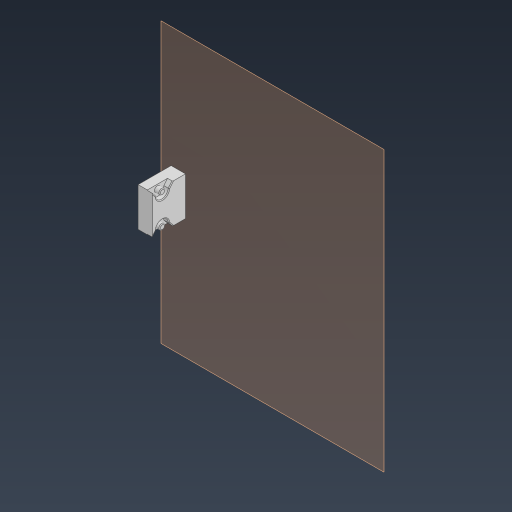
# Autodesk Inventor part: front-lunad-holder
Saved by Autodesk Inventor 2023 (Build 270158000, 158)
## iProperties
Created: 2025-04-06
Part Number: front-lunad-holder
Material: Generic
Document SubType Name: Modeling
Designer: szymo
Density: 1 g/cm^3
Appearance: Default
Author: szymo
Autodesk Inventor part; units mm, degrees
ref_plane "YZ Plane" through (0, 0, 0) normal (1, 0, 0) x (0, 1, 0)
ref_plane "XZ Plane" through (0, 0, 0) normal (0, 1, 0) x (-1, 0, 0)
ref_plane "XY Plane" through (0, 0, 0) normal (0, 0, 1) x (1, 0, 0)
ref_plane "Work Plane1" through (0, 0, 0) normal (0, 0, 1) x (1, 0, 0)
sketch "Sketch1" plane through (0, 0, 0) normal (0, 0, 1) x (1, 0, 0)
  line L0 (-33.9, 7.85) -> (-44.9, 7.85) projected
  line L1 (-35.9, 5.925) -> (-35.9, 7.85) projected
  line L2 (-35.9, 5.925) -> (-35.9, 3.675) projected
  line L3 (-35.9, -7.85) -> (-35.9, -5.925) projected
  line L4 (-35.9, -3.675) -> (-35.9, -5.925) projected
  line L5 (-44.9, -7.85) -> (-33.9, -7.85) projected
  line L6 (-33.9, 7.55) -> (-44.9, 7.55)
  line L7 (-44.9, -7.55) -> (-33.9, -7.55)
  line L8 (-39.5, 49.5) -> (-39.5, -49.5) projected
  line L9 (-39.5, 7.55) -> (-39.5, -7.55)
  line L10 (-33.9, 5.925) -> (-33.9, 3.675) projected
  line L11 (-33.9, 5.925) -> (-33.9, 7.85) projected
  line L12 (-35.9, 3.675) -> (-33.9, 3.675)
  line L13 (-33.9, -7.85) -> (-33.9, -5.925) projected
  line L14 (-33.9, -3.675) -> (-33.9, -5.925) projected
  line L15 (-35.9, -3.675) -> (-33.9, -3.675)
  line L16 (-33.9, 3.675) -> (-33.9, -3.675)
  line L17 (-35.9, -3.675) -> (-35.9, 3.675)
  point P0 (0, 0)
  dimension "d0" = 0.3
  dimension "d1" = 0.3
  constraints: 14 end point, 4 point on line, 3 parallel, 2 horizontal, 1 collinear
  measures "d0" distance between parallel lines of L0 L6
  measures "d1" distance between parallel lines of L5 L7
extrude "Extrusion1" add sketch "Sketch1" along normal up to surface (12.8653 mm away) contours L11 L10 L12 L2 L1 L6 | L1 L2 L17 L4 L3 L7 L8 L6 | L16 L15 L17 L12 | L14 L13 L7 L3 L4 L15
sketch "Sketch2" plane through (-33.9, -7.55, 0) normal (1, 0, 0) x (0, 0, -1)
  arc A0 (-6.75, 1.625) -> (-11.25, 1.625) centre (-9, 1.625) ccw projected
  line L0 (-12.8653, -0.3) -> (-11.25, 1.625) projected
  line L1 (-6.75, 1.625) -> (-5.1347, -0.3) projected
  line L2 (-5.1347, 15.4) -> (-6.75, 13.475) projected
  arc A1 (-11.25, 13.475) -> (-6.75, 13.475) centre (-9, 13.475) ccw projected
  line L3 (-11.25, 13.475) -> (-12.8653, 15.4) projected
  line L4 (-12.8653, 15.1) -> (-12.8653, 0) projected
  line L5 (0, 0) -> (-12.8653, 0) projected
  line L6 (0, 0) -> (0, 15.1) projected
  line L7 (0, 15.1) -> (-12.8653, 15.1) projected
  line L8 (-13.0951, -0.1072) -> (-11.5475, 1.7371)
  arc A2 (-6.4525, 1.7371) -> (-11.5475, 1.7371) centre (-9, 1.625) ccw
  line L9 (-6.4525, 1.7371) -> (-4.9049, -0.1072)
  line L10 (-4.9049, 15.2072) -> (-6.4525, 13.3629)
  arc A3 (-11.5475, 13.3629) -> (-6.4525, 13.3629) centre (-9, 13.475) ccw
  line L11 (-11.5475, 13.3629) -> (-13.0951, 15.2072)
  circle A4 centre (-9, 1.625) radius 1.1 projected
  circle A5 centre (-9, 13.475) radius 1.1 projected
  circle A6 centre (-9, 1.625) radius 1
  circle A7 centre (-9, 13.475) radius 1
  point P0 (0, 7.55)
  point P1 (-12.8653, 14.9333)
  point P2 (-4.9948, 15.1)
  point P3 (-4.9948, 0)
  point P4 (-12.8653, 0.1667)
  dimension "d4" = 0.3
  dimension "d5" = 0.3
  dimension "d6" = 0.1
  dimension "d7" = 0.1
  constraints: 8 end point, 4 centre point, 4 point on circle, 4 other
  measures "d4" radial gap between concentric circles of A0 A2
  measures "d5" radial gap between concentric circles of A1 A3
  measures "d6" radial gap between concentric circles of A4 A6
  measures "d7" radial gap between concentric circles of A5 A7
extrude "Extrusion2" cut sketch "Sketch2" against normal blind 2 contours L1 L5 L0 A0 | A0 L0 L5 L4 L8 A2 L9 L1 | L4 L7 L3 A1 L2 L10 A3 L11 | L2 A1 L3 L7
fillet "Fillet1" radius 0.3 8 edges at (-33.9, -5.925, 10.1) (-33.9, 5.925, 10.1) (-33.9, -6.5981, 12.2064) (-33.9, -3.375, 9) (-33.9, -6.6814, 5.7237) (-33.9, 6.6814, 5.7237) (-33.9, 6.5981, 12.2064) (-33.9, 3.375, 9)
sketch "Sketch3" plane through (0, 0, 0) normal (0, 0, -1) x (-1, 0, 0)
  line L0 (33.9, -7.55) -> (33.9, 7.55) projected
  line L1 (39.5, -7.55) -> (33.9, -7.55) projected
  line L2 (39.5, 7.55) -> (39.5, -7.55) projected
  line L3 (33.9, 7.55) -> (39.5, 7.55) projected
  line L4 (33.9, 6.9166) -> (33.9, -6.9166) projected
  line L5 (33.9, 0) -> (39.5, 0) construction
  line L6 (33.9, -7.55) -> (39.5, 0) construction
  line L7 (33.9, 0) -> (39.5, -7.55) construction
  line L8 (39.5, 0) -> (33.9, 7.55) construction
  line L9 (39.5, 7.55) -> (33.9, 0) construction
  point P0 (0, 0)
  point P1 (36.7, -3.775)
  point P2 (36.7, 3.775)
  constraints: 10 end point, 4 midpoint, 2 parallel
hole "Hole1" at (-36.7, -3.775, 0) at (-36.7, 3.775, 0) direction (0, 0, 1) diameter 4 depth 4.5 counterbore diameter 5 counterbore depth 0.5
body "Solid1"
